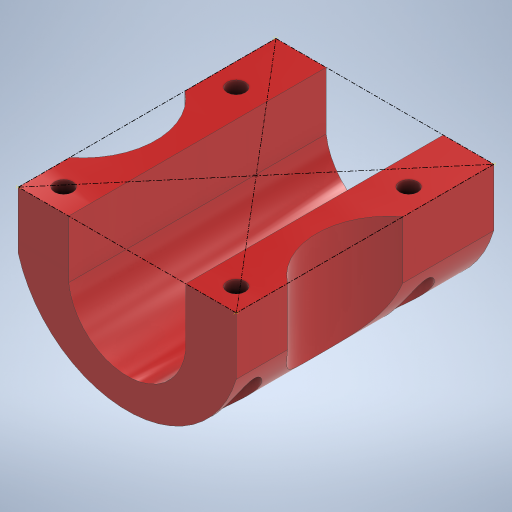
# Autodesk Inventor part: XZ_Side_Belt
Saved by Autodesk Inventor 2023 (Build 270158000, 158)
## iProperties
Created: 2023-11-25
Part Number: XZ_Side_Belt
Material: Generic
Document SubType Name: Modeling
Designer: danie
Density: 1 g/cm^3
Appearance: Default
Author: danie
Autodesk Inventor part; units mm, degrees
ref_plane "YZ Plane" through (0, 0, 0) normal (1, 0, 0) x (0, 1, 0)
ref_plane "XY Plane" through (0, 0, 0) normal (0, 0, 1) x (1, 0, 0)
sketch "Sketch1" plane through (0, 0, 0) normal (0, 0, 1) x (1, 0, 0)
  line L0 (78.5, 134.5339) -> (78.5, 141.8499) projected
  line L1 (89.6, 141.8499) -> (89.6, 134.5339) projected
  line L2 (78.5, 129.1499) -> (78.5, 134.5339) projected
  line L3 (115.4, 134.5339) -> (115.4, 141.8499) projected
  line L4 (115.4, 141.8499) -> (126.5, 141.8499) projected
  line L5 (78.5, 141.8499) -> (89.6, 141.8499) projected
  line L6 (126.5, 141.8499) -> (126.5, 134.5339) projected
  line L7 (126.5, 134.5339) -> (126.5, 129.1499) projected
  line L8 (89.6, 134.5339) -> (89.6, 129.1499) projected
  line L9 (89.6, 129.1499) -> (115.4, 129.1499)
  line L10 (115.4, 129.1499) -> (115.4, 134.5339)
  line L11 (89.6, 134.5339) -> (89.6, 129.1499)
  arc A0 (89.6, 129.1499) -> (115.4, 129.1499) centre (102.5, 130.7593) ccw
  arc A1 (78.5, 129.1499) -> (126.5, 129.1499) centre (102.5, 136.1499) ccw
  point P0 (0, 0)
  dimension "d0" = 13
  dimension "d1" = 25
  constraints: 6 end point, 4 point on circle, 2 centre point, 1 horizontal, 1 parallel, 1 perpendicular
  measures "d0" radius of A0
  measures "d1" radius of A1
sketch "Sketch2" plane through (0, 0, 0) normal (0, 1, 0) x (-1, 0, 0)
  line L0 (-78.5, 20.0189) -> (-78.5, 0)
  line L1 (-78.5, 0) -> (-126.5, 0)
  line L2 (-126.5, 0) -> (-126.5, 20.0189)
  line L3 (-126.5, 20.0189) -> (-126.5, 45.4189)
  line L4 (-126.5, 45.4189) -> (-126.5, 56.7189)
  line L5 (-126.5, 56.7189) -> (-78.5, 56.7189)
  line L6 (-78.5, 56.7189) -> (-78.5, 45.4189)
  line L7 (-78.5, 45.4189) -> (-78.5, 20.0189)
  arc A0 (-78.5, 45.4189) -> (-78.5, 20.0189) centre (-68.7681, 32.7189) ccw
  arc A1 (-126.5, 20.0189) -> (-126.5, 45.4189) centre (-136.2319, 32.7189) ccw
  circle A2 centre (-83.4998, 51.7195) radius 2.0243 projected
  circle A3 centre (-121.5027, 51.7228) radius 2.0203 projected
  circle A4 centre (-121.4978, 13.7152) radius 2.0293 projected
  circle A5 centre (-83.5003, 13.7201) radius 2.0237 projected
  point P0 (0, 0)
  dimension "d2" = 16
  dimension "d3" = 16
  constraints: 16 end point, 4 coincident, 4 perpendicular, 4 point on circle, 3 collinear, 2 centre point, 1 vertical
  measures "d2" radius of A0
  measures "d3" radius of A1
extrude "Extrusion1" add sketch "Sketch1" along normal blind 60 contours L0 L5 L1 L8 A0 L10 L3 L4 L6 L7 A1 L2
extrude "Extrusion2" cut sketch "Sketch2" along normal up to surface (141.8499 mm away) contours L0 L1 L2 A1 L4 L5 L6 A0 | A2 | A3 | A4 | A5 keep common part
ref_plane "Work Plane1" through (126.082, 127.8499, 56.7189) normal (0, 1, 0) x (-1, 0, 0)
ref_plane "Work Plane3" through (89.6, 141.8499, 56.7189) normal (0, 1, 0) x (1, 0, 0)
sketch "Sketch5" plane through (89.6, 141.8499, 56.7189) normal (0, 1, 0) x (1, 0, 0)
  line L0 (-11.1, 0) -> (36.9, 56.7189)
  line L1 (0, 56.7189) -> (-11.1, 56.7189) projected
  line L2 (36.9, 0) -> (-11.1, 56.7189)
  line L3 (36.9, 11.3) -> (36.9, 0) projected
  line L4 (36.9, 0) -> (-11.1, 0)
  line L5 (-11.1, 0) -> (-11.1, 56.7189)
  line L6 (-11.1, 56.7189) -> (36.9, 56.7189)
  line L7 (36.9, 56.7189) -> (36.9, 0)
  point P0 (12.9, 28.3595)
  constraints: 12 end point, 2 parallel, 1 horizontal, 1 midpoint, 1 perpendicular
sketch "Sketch6" plane through (0, 0, 0) normal (0, 1, 0) x (-1, 0, 0)
  arc A0 (-126.5, 20.0189) -> (-126.5, 45.4189) centre (-136.2319, 32.7189) ccw projected
  line L0 (-126.5, 0) -> (-126.5, 20.0189) projected
  line L1 (-126.5, 0) -> (-115.4, 0) projected
  line L2 (-115.4, 0) -> (-115.4, 56.7189) projected
  line L3 (-126.5, 56.7189) -> (-115.4, 56.7189) projected
  line L4 (-126.5, 45.4189) -> (-126.5, 56.7189) projected
  arc A1 (-78.5, 45.4189) -> (-78.5, 20.0189) centre (-68.7681, 32.7189) ccw projected
  line L5 (-78.5, 45.4189) -> (-78.5, 56.7189) projected
  line L6 (-89.6, 56.7189) -> (-78.5, 56.7189) projected
  line L7 (-89.6, 0) -> (-89.6, 56.7189) projected
  line L8 (-89.6, 0) -> (-78.5, 0) projected
  line L9 (-78.5, 0) -> (-78.5, 20.0189) projected
  line L10 (-78.5, 56.7189) -> (-126.5, 56.7189)
  line L11 (-126.5, 56.7189) -> (-126.5, 8.7189)
  line L12 (-126.5, 8.7189) -> (-78.5, 8.7189)
  line L13 (-78.5, 8.7189) -> (-78.5, 56.7189)
  line L14 (-78.5, 8.7189) -> (-126.5, 56.7189)
  line L15 (-78.5, 56.7189) -> (-126.5, 8.7189)
  line L16 (-83.5, 13.7189) -> (-121.5, 13.7189)
  line L17 (-121.5, 13.7189) -> (-121.5, 51.7189)
  line L18 (-121.5, 51.7189) -> (-83.5, 51.7189)
  line L19 (-83.5, 51.7189) -> (-83.5, 13.7189)
  line L20 (-83.5, 13.7189) -> (-121.5, 51.7189) construction
  line L21 (-121.5, 13.7189) -> (-83.5, 51.7189) construction
  circle A2 centre (-83.5, 13.7189) radius 4
  circle A3 centre (-83.5, 51.7189) radius 4
  circle A4 centre (-121.5, 51.7189) radius 4
  circle A5 centre (-121.5, 13.7189) radius 4
  point P0 (0, 0)
  point P1 (-102.5, 32.7189)
  dimension "d21" = 48
  dimension "d22" = 38
  dimension "d23" = 38
  dimension "d24" = 8
  dimension "d25" = 8
  dimension "d26" = 8
  dimension "d27" = 8
  constraints: 24 end point, 4 centre point, 4 coincident, 4 parallel, 3 midpoint, 2 horizontal, 2 perpendicular, 1 point on line
  measures "d21" distance of L11.end L10.end
  measures "d22" distance of L17.end L18.end
  measures "d23" distance of L16.end L17.end
  measures "d24" diameter of A2
  measures "d25" diameter of A3
  measures "d26" diameter of A4
  measures "d27" diameter of A5
extrude "Extrusion4" cut sketch "Sketch6" along normal up to surface (129.1499 mm away) contours A5 L15 L17 | L17 L15 A5 | L15 L16 A5 | A4 L14 L17 | L17 L14 A4 | L15 A5 L16 | A4 L18 L14 | L18 A4 L14 | A2 L14 L16 | L16 L14 A2 | L14 L19 A2 | A2 L19 L14 | A3 L15 L18 | L18 L15 A3 | A3 L19 L15 | L15 L19 A3
sketch "Sketch7" plane through (121.5, 129.1499, 13.7189) normal (0, -1, 0) x (1, 0, 0)
  circle A0 centre (0, 0) radius 4 projected
  circle A1 centre (-38, 0) radius 4 projected
  circle A2 centre (-38, 38) radius 4 projected
  circle A3 centre (0, 38) radius 4 projected
  point P0 (-121.5, -13.7189)
hole "Hole2" at (121.5, 129.1499, 13.7189) at (121.5, 129.1499, 51.7189) at (83.5, 129.1499, 51.7189) at (83.5, 129.1499, 13.7189) direction (0, 1, 0) diameter 4 end through all clearance for "Slotted Cheese Head Screw ISO 1207" size "M4" standard "ISO"
body "Solid1"
